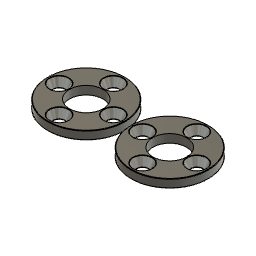
ShockPiston 2mm (Autodesk Fusion 360 design; units mm, degrees)
Autodesk Fusion 360 part; units mm, degrees
sketch "Sketch1" plane through (0, 0, 0) normal (0, 1, 0) x (1, 0, 0)
  circle A0 centre (0, 0) radius 9.25
  line L0 (0, 0) -> (0, 6.5) construction
  line L1 (0, 0) -> (-6.5, 0) construction
  line L2 (0, 0) -> (0, -6.5) construction
  line L3 (0, 0) -> (6.5, 0) construction
  circle A1 centre (-6.5, 0) radius 1.3505
  circle A2 centre (6.5, 0) radius 1.3505
  circle A3 centre (0, -6.5) radius 1.3505
  circle A4 centre (0, 6.5) radius 1.3505
  circle A5 centre (0, 0) radius 4.025
  dimension "d2" = 6.5
  dimension "d13" = 18.5
  dimension "d14" = 8.05
  constraint coincident A0.centre L0.start
  constraint perpendicular L0 L1
  constraint perpendicular L1 L2
  constraint perpendicular L2 L3
  constraint equal L0 L1
  constraint equal L1 L2
  constraint equal L1 L3
  constraint coincident L1.end A1.centre
  constraint coincident L3.end A2.centre
  constraint coincident L2.end A3.centre
  constraint coincident L0.end A4.centre
  constraint equal A1 A4
  constraint equal A1 A3
  constraint equal A1 A2
  measures "d2" distance of A0.centre L1.end
  measures "d13" diameter of A0
  measures "d14" diameter of A5
extrude "Extrude2" add sketch "Sketch1" along normal blind 2 makes body 1
extrude "Extrude3" cut sketch "Sketch1" along normal blind 2 draft 25 contours A1 | A2 | A3 | A4 bodies 1
fillet "Fillet2" radius 0.1 1 edges at (-2.1286, 2, 5.6744) 4 faces at (1.5217, 1.5556, -7.912) (-6.0381, 1.5556, 2.0238) (1.8703, 1.5556, 7.4007) (6.9619, 1.5556, 2.0238) on bodies 1
fillet "Fillet3" radius 0.1 1 faces at (9.2385, 1.3333, 0.4611) on bodies 1
copy_body "CopyPasteBodies2" bodies 1 makes body 2
move_body "Move3" bodies 2 to x (1, 0, 0) y (0, 1, 0) z (0, 0, 1) at (20, 0, 0)
